Autodesk Fusion 360 part; units mm, degrees
(part 6 of 18)
  spline S29 degree 5 poles (33.0522, -6.0428) (33.0487, -6.0404) (33.0419, -6.0356) (33.0316, -6.0284) (33.018, -6.0188) (33.0009, -6.0069) (32.9839, -5.995) (32.9669, -5.9831) (32.9499, -5.9714) (32.9329, -5.9596) (32.9159, -5.948) (32.899, -5.9363) (32.8821, -5.9248) (32.8652, -5.9132) (32.8483, -5.9018) (32.8314, -5.8903) (32.8145, -5.879) (32.7977, -5.8676) (32.7809, -5.8563) (32.7641, -5.8451) (32.7473, -5.8339) (32.7306, -5.8228) (32.7138, -5.8117) (32.6971, -5.8007) (32.6804, -5.7897) (32.6637, -5.7788) (32.6471, -5.7679) (32.6305, -5.7571) (32.6139, -5.7463) (32.5973, -5.7356) (32.5807, -5.7249) (32.5642, -5.7143) (32.5476, -5.7037) (32.5311, -5.6932) (32.5147, -5.6827) (32.4982, -5.6723) (32.4818, -5.6619) (32.4654, -5.6516) (32.449, -5.6413) (32.4326, -5.6311) (32.4163, -5.6209) (32.4, -5.6108) (32.3837, -5.6007) (32.3675, -5.5907) (32.3512, -5.5807) (32.335, -5.5708) (32.3188, -5.5609) (32.3027, -5.5511) (32.2865, -5.5414) (32.2704, -5.5316) (32.2544, -5.522) (32.2383, -5.5123) (32.2223, -5.5028) (32.2063, -5.4933) (32.1903, -5.4838) (32.1744, -5.4744) (32.1585, -5.465) (32.1426, -5.4557) (32.1267, -5.4464) (32.1109, -5.4372) (32.0951, -5.4281) (32.0793, -5.419) (32.0636, -5.4099) (32.0479, -5.4009) (32.0322, -5.3919) (32.0166, -5.383) (32.0009, -5.3742) (31.9854, -5.3654) (31.9698, -5.3566) (31.9543, -5.3479) (31.9388, -5.3393) (31.9233, -5.3307) (31.9079, -5.3221) (31.8925, -5.3136) (31.8771, -5.3052) (31.8618, -5.2968) (31.8465, -5.2884) (31.8313, -5.2801) (31.816, -5.2719) (31.8008, -5.2637) (31.7857, -5.2555) (31.7706, -5.2474) (31.7555, -5.2394) (31.7404, -5.2314) (31.7254, -5.2235) (31.7104, -5.2156) (31.6955, -5.2077) (31.6806, -5.2) (31.6657, -5.1922) (31.6509, -5.1845) (31.6361, -5.1769) (31.6213, -5.1693) (31.6066, -5.1618) (31.5919, -5.1543) (31.5773, -5.1469) (31.5627, -5.1395) (31.5481, -5.1322) (31.5336, -5.1249) (31.5191, -5.1177) (31.5047, -5.1105) (31.4903, -5.1034) (31.4759, -5.0963) (31.4616, -5.0893) (31.4474, -5.0823) (31.4331, -5.0754) (31.419, -5.0686) (31.4048, -5.0617) (31.3907, -5.055) (31.3767, -5.0483) (31.3627, -5.0416) (31.3487, -5.035) (31.3348, -5.0284) (31.3209, -5.0219) (31.3071, -5.0155) (31.2933, -5.0091) (31.2796, -5.0027) (31.2659, -4.9964) (31.2522, -4.9902) (31.2387, -4.984) (31.2251, -4.9778) (31.2116, -4.9717) (31.1982, -4.9657) (31.1848, -4.9597) (31.1714, -4.9537) (31.1582, -4.9478) (31.1449, -4.942) (31.1317, -4.9362) (31.1186, -4.9305) (31.1055, -4.9248) (31.0925, -4.9191) (31.0795, -4.9136) (31.0666, -4.908) (31.0537, -4.9025) (31.0409, -4.8971) (31.0281, -4.8917) (31.0154, -4.8864) (31.0028, -4.8811) (30.9902, -4.8759) (30.9777, -4.8707) (30.9652, -4.8656) (30.9528, -4.8605) (30.9405, -4.8555) (30.9282, -4.8505) (30.9159, -4.8456) (30.9038, -4.8407) (30.8916, -4.8359) (30.8796, -4.8311) (30.8676, -4.8264) (30.8557, -4.8217) (30.8438, -4.8171) (30.832, -4.8126) (30.8203, -4.808) (30.8086, -4.8036) (30.797, -4.7992) (30.7855, -4.7948) (30.774, -4.7905) (30.7626, -4.7862) (30.7513, -4.782) (30.7401, -4.7779) (30.7289, -4.7738) (30.7178, -4.7697) (30.7067, -4.7657) (30.6957, -4.7617) (30.6848, -4.7578) (30.674, -4.754) (30.6633, -4.7502) (30.6526, -4.7464) (30.642, -4.7427) (30.6315, -4.7391) (30.621, -4.7354) (30.6106, -4.7319) (30.6004, -4.7284) (30.5901, -4.7249) (30.58, -4.7215) (30.57, -4.7182) (30.56, -4.7149) (30.5501, -4.7116) (30.5403, -4.7084) (30.5306, -4.7053) (30.521, -4.7022) (30.5115, -4.6991) (30.502, -4.6961) (30.4926, -4.6932) (30.4834, -4.6903) (30.4742, -4.6874) (30.4651, -4.6846) (30.4561, -4.6818) (30.4472, -4.6791) (30.4384, -4.6765) (30.4297, -4.6739) (30.4211, -4.6713) (30.4126, -4.6688) (30.4042, -4.6663) (30.3958, -4.6639) (30.3876, -4.6616) (30.3795, -4.6593) (30.3715, -4.657) (30.3636, -4.6548) (30.3559, -4.6526) (30.3482, -4.6505) (30.3406, -4.6484) (30.3332, -4.6464) (30.3258, -4.6444) (30.3186, -4.6425) (30.3115, -4.6407) (30.3045, -4.6388) (30.2976, -4.637) (30.2909, -4.6353) (30.2842, -4.6336) (30.2777, -4.632) (30.2713, -4.6304) (30.2651, -4.6289) (30.259, -4.6274) (30.253, -4.6259) (30.2471, -4.6245) (30.2414, -4.6232) (30.2358, -4.6219) (30.2304, -4.6206) (30.2251, -4.6194) (30.22, -4.6182) (30.215, -4.6171) (30.2101, -4.6161) (30.2054, -4.615) (30.2009, -4.614) (30.1965, -4.6131) (30.1923, -4.6122) (30.1882, -4.6114) (30.1843, -4.6106) (30.1806, -4.6098) (30.1771, -4.6091) (30.1737, -4.6084) (30.1705, -4.6078) (30.1675, -4.6072) (30.1647, -4.6067) (30.162, -4.6062) (30.1596, -4.6058) (30.1574, -4.6054) (30.1553, -4.605) (30.1535, -4.6047) (30.1519, -4.6044) (30.1505, -4.6042) (30.1496, -4.604) (30.149, -4.6039) (30.1487, -4.6039) (30.1485, -4.6039) knots -1 -1 -1 -1 -1 -1 -0.99583333 -0.99166667 -0.9875 -0.98333333 -0.97916667 -0.975 -0.97083333 -0.96666667 -0.9625 -0.95833333 -0.95416667 -0.95 -0.94583333 -0.94166667 -0.9375 -0.93333333 -0.92916667 -0.925 -0.92083333 -0.91666667 -0.9125 -0.90833333 -0.90416667 -0.9 -0.89583333 -0.89166667 -0.8875 -0.88333333 -0.87916667 -0.875 -0.87083333 -0.86666667 -0.8625 -0.85833333 -0.85416667 -0.85 -0.84583333 -0.84166667 -0.8375 -0.83333333 -0.82916667 -0.825 -0.82083333 -0.81666667 -0.8125 -0.80833333 -0.80416667 -0.8 -0.79583333 -0.79166667 -0.7875 -0.78333333 -0.77916667 -0.775 -0.77083333 -0.76666667 -0.7625 -0.75833333 -0.75416667 -0.75 -0.74583333 -0.74166667 -0.7375 -0.73333333 -0.72916667 -0.725 -0.72083333 -0.71666667 -0.7125 -0.70833333 -0.70416667 -0.7 -0.69583333 -0.69166667 -0.6875 -0.68333333 -0.67916667 -0.675 -0.67083333 -0.66666667 -0.6625 -0.65833333 -0.65416667 -0.65 -0.64583333 -0.64166667 -0.6375 -0.63333333 -0.62916667 -0.625 -0.62083333 -0.61666667 -0.6125 -0.60833333 -0.60416667 -0.6 -0.59583333 -0.59166667 -0.5875 -0.58333333 -0.57916667 -0.575 -0.57083333 -0.56666667 -0.5625 -0.55833333 -0.55416667 -0.55 -0.54583333 -0.54166667 -0.5375 -0.53333333 -0.52916667 -0.525 -0.52083333 -0.51666667 -0.5125 -0.50833333 -0.50416667 -0.5 -0.49583333 -0.49166667 -0.4875 -0.48333333 -0.47916667 -0.475 -0.47083333 -0.46666667 -0.4625 -0.45833333 -0.45416667 -0.45 -0.44583333 -0.44166667 -0.4375 -0.43333333 -0.42916667 -0.425 -0.42083333 -0.41666667 -0.4125 -0.40833333 -0.40416667 -0.4 -0.39583333 -0.39166667 -0.3875 -0.38333333 -0.37916667 -0.375 -0.37083333 -0.36666667 -0.3625 -0.35833333 -0.35416667 -0.35 -0.34583333 -0.34166667 -0.3375 -0.33333333 -0.32916667 -0.325 -0.32083333 -0.31666667 -0.3125 -0.30833333 -0.30416667 -0.3 -0.29583333 -0.29166667 -0.2875 -0.28333333 -0.27916667 -0.275 -0.27083333 -0.26666667 -0.2625 -0.25833333 -0.25416667 -0.25 -0.24583333 -0.24166667 -0.2375 -0.23333333 -0.22916667 -0.225 -0.22083333 -0.21666667 -0.2125 -0.20833333 -0.20416667 -0.2 -0.19583333 -0.19166667 -0.1875 -0.18333333 -0.17916667 -0.175 -0.17083333 -0.16666667 -0.1625 -0.15833333 -0.15416667 -0.15 -0.14583333 -0.14166667 -0.1375 -0.13333333 -0.12916667 -0.125 -0.12083333 -0.11666667 -0.1125 -0.10833333 -0.10416667 -0.1 -0.09583333 -0.09166667 -0.0875 -0.08333333 -0.07916667 -0.075 -0.07083333 -0.06666667 -0.0625 -0.05833333 -0.05416667 -0.05 -0.04583333 -0.04166667 -0.0375 -0.03333333 -0.02916667 -0.025 -0.02083333 -0.01666667 -0.0125 -0.00833333 -0.00416667 0 0 0 0 0 0
  line L58 (30.1485, -4.6039) -> (30.1472, -4.6036)
  line L59 (30.1472, -4.6036) -> (28.5441, -4.3588)
  arc A30 (28.5441, -4.3588) -> (28.8266, -1.6711) centre (0, 0) ccw
  line L60 (28.8266, -1.6711) -> (30.4455, -1.7649)
  line L61 (30.4455, -1.7649) -> (30.4469, -1.765)
  spline S30 degree 5 poles (30.4469, -1.765) (30.4471, -1.765) (30.4474, -1.765) (30.448, -1.765) (30.449, -1.7651) (30.4503, -1.7651) (30.452, -1.7652) (30.4538, -1.7653) (30.4559, -1.7653) (30.4581, -1.7654) (30.4606, -1.7655) (30.4633, -1.7655) (30.4662, -1.7656) (30.4692, -1.7657) (30.4725, -1.7657) (30.4759, -1.7658) (30.4795, -1.7658) (30.4833, -1.7658) (30.4873, -1.7659) (30.4914, -1.7659) (30.4958, -1.7659) (30.5002, -1.7659) (30.5049, -1.7659) (30.5097, -1.7659) (30.5147, -1.7658) (30.5198, -1.7658) (30.5251, -1.7657) (30.5305, -1.7656) (30.5361, -1.7655) (30.5418, -1.7654) (30.5477, -1.7653) (30.5537, -1.7651) (30.5598, -1.7649) (30.5661, -1.7647) (30.5726, -1.7645) (30.5791, -1.7643) (30.5858, -1.7641) (30.5927, -1.7638) (30.5996, -1.7635) (30.6067, -1.7632) (30.6139, -1.7629) (30.6213, -1.7625) (30.6288, -1.7621) (30.6363, -1.7617) (30.6441, -1.7613) (30.6519, -1.7609) (30.6598, -1.7604) (30.6679, -1.7599) (30.6761, -1.7594) (30.6844, -1.7588) (30.6928, -1.7582) (30.7013, -1.7576) (30.7099, -1.757) (30.7187, -1.7563) (30.7275, -1.7557) (30.7365, -1.755) (30.7455, -1.7542) (30.7547, -1.7534) (30.764, -1.7527) (30.7734, -1.7518) (30.7828, -1.751) (30.7924, -1.7501) (30.8021, -1.7492) (30.8118, -1.7482) (30.8217, -1.7473) (30.8317, -1.7463) (30.8417, -1.7452) (30.8519, -1.7442) (30.8621, -1.7431) (30.8725, -1.7419) (30.8829, -1.7408) (30.8934, -1.7396) (30.904, -1.7384) (30.9148, -1.7371) (30.9255, -1.7358) (30.9364, -1.7345) (30.9474, -1.7331) (30.9584, -1.7318) (30.9696, -1.7303) (30.9808, -1.7289) (30.9921, -1.7274) (31.0035, -1.7259) (31.015, -1.7243) (31.0265, -1.7227) (31.0382, -1.7211) (31.0499, -1.7195) (31.0617, -1.7178) (31.0736, -1.716) (31.0855, -1.7143) (31.0976, -1.7125) (31.1097, -1.7106) (31.1219, -1.7088) (31.1341, -1.7069) (31.1465, -1.7049) (31.1589, -1.7029) (31.1714, -1.7009) (31.1839, -1.6989) (31.1965, -1.6968) (31.2092, -1.6947) (31.222, -1.6925) (31.2349, -1.6903) (31.2478, -1.6881) (31.2608, -1.6858) (31.2738, -1.6835) (31.287, -1.6812) (31.3002, -1.6788) (31.3134, -1.6763) (31.3268, -1.6739) (31.3402, -1.6714) (31.3536, -1.6689) (31.3672, -1.6663) (31.3808, -1.6637) (31.3944, -1.661) (31.4081, -1.6583) (31.4219, -1.6556) (31.4358, -1.6528) (31.4497, -1.65) (31.4637, -1.6472) (31.4777, -1.6443) (31.4918, -1.6414) (31.506, -1.6384) (31.5202, -1.6354) (31.5345, -1.6324) (31.5488, -1.6293) (31.5632, -1.6262) (31.5777, -1.623) (31.5922, -1.6198) (31.6068, -1.6166) (31.6215, -1.6133) (31.6362, -1.61) (31.6509, -1.6066) (31.6657, -1.6032) (31.6806, -1.5998) (31.6955, -1.5963) (31.7105, -1.5928) (31.7255, -1.5892) (31.7406, -1.5856) (31.7557, -1.582) (31.7709, -1.5783) (31.7862, -1.5746) (31.8015, -1.5708) (31.8168, -1.567) (31.8322, -1.5632) (31.8477, -1.5593) (31.8632, -1.5553) (31.8788, -1.5514) (31.8944, -1.5473) (31.9101, -1.5433) (31.9258, -1.5392) (31.9415, -1.5351) (31.9573, -1.5309) (31.9732, -1.5267) (31.9891, -1.5224) (32.0051, -1.5181) (32.0211, -1.5137) (32.0372, -1.5093) (32.0533, -1.5049) (32.0694, -1.5004) (32.0856, -1.4959) (32.1019, -1.4914) (32.1181, -1.4868) (32.1345, -1.4821) (32.1509, -1.4774) (32.1673, -1.4727) (32.1838, -1.4679) (32.2003, -1.4631) (32.2169, -1.4583) (32.2335, -1.4534) (32.2501, -1.4484) (32.2668, -1.4434) (32.2836, -1.4384) (32.3003, -1.4333) (32.3172, -1.4282) (32.334, -1.4231) (32.3509, -1.4179) (32.3679, -1.4126) (32.3849, -1.4073) (32.4019, -1.402) (32.419, -1.3966) (32.4361, -1.3912) (32.4533, -1.3858) (32.4705, -1.3803) (32.4877, -1.3747) (32.505, -1.3691) (32.5223, -1.3635) (32.5397, -1.3578) (32.5571, -1.3521) (32.5745, -1.3463) (32.592, -1.3405) (32.6095, -1.3347) (32.627, -1.3288) (32.6446, -1.3228) (32.6622, -1.3169) (32.6799, -1.3108) (32.6976, -1.3048) (32.7153, -1.2986) (32.7331, -1.2925) (32.7509, -1.2863) (32.7688, -1.28) (32.7867, -1.2738) (32.8046, -1.2674) (32.8225, -1.261) (32.8405, -1.2546) (32.8585, -1.2482) (32.8766, -1.2416) (32.8947, -1.2351) (32.9128, -1.2285) (32.931, -1.2218) (32.9492, -1.2152) (32.9674, -1.2084) (32.9856, -1.2016) (33.0039, -1.1948) (33.0223, -1.188) (33.0406, -1.181) (33.059, -1.1741) (33.0774, -1.1671) (33.0959, -1.16) (33.1144, -1.153) (33.1329, -1.1458) (33.1514, -1.1387) (33.17, -1.1314) (33.1886, -1.1242) (33.2073, -1.1168) (33.2259, -1.1095) (33.2447, -1.1021) (33.2634, -1.0946) (33.2821, -1.0872) (33.3009, -1.0796) (33.3198, -1.072) (33.3386, -1.0644) (33.3575, -1.0567) (33.3764, -1.049) (33.3953, -1.0413) (33.4143, -1.0335) (33.4333, -1.0256) (33.4523, -1.0177) (33.4714, -1.0098) (33.4904, -1.0018) (33.5096, -0.9938) (33.5287, -0.9857) (33.5478, -0.9776) (33.5632, -0.971) (33.5747, -0.9661) (33.5824, -0.9628) (33.5862, -0.9612) knots 0 0 0 0 0 0 0.00416667 0.00833333 0.0125 0.01666667 0.02083333 0.025 0.02916667 0.03333333 0.0375 0.04166667 0.04583333 0.05 0.05416667 0.05833333 0.0625 0.06666667 0.07083333 0.075 0.07916667 0.08333333 0.0875 0.09166667 0.09583333 0.1 0.10416667 0.10833333 0.1125 0.11666667 0.12083333 0.125 0.12916667 0.13333333 0.1375 0.14166667 0.14583333 0.15 0.15416667 0.15833333 0.1625 0.16666667 0.17083333 0.175 0.17916667 0.18333333 0.1875 0.19166667 0.19583333 0.2 0.20416667 0.20833333 0.2125 0.21666667 0.22083333 0.225 0.22916667 0.23333333 0.2375 0.24166667 0.24583333 0.25 0.25416667 0.25833333 0.2625 0.26666667 0.27083333 0.275 0.27916667 0.28333333 0.2875 0.29166667 0.29583333 0.3 0.30416667 0.30833333 0.3125 0.31666667 0.32083333 0.325 0.32916667 0.33333333 0.3375 0.34166667 0.34583333 0.35 0.35416667 0.35833333 0.3625 0.36666667 0.37083333 0.375 0.37916667 0.38333333 0.3875 0.39166667 0.39583333 0.4 0.40416667 0.40833333 0.4125 0.41666667 0.42083333 0.425 0.42916667 0.43333333 0.4375 0.44166667 0.44583333 0.45 0.45416667 0.45833333 0.4625 0.46666667 0.47083333 0.475 0.47916667 0.48333333 0.4875 0.49166667 0.49583333 0.5 0.50416667 0.50833333 0.5125 0.51666667 0.52083333 0.525 0.52916667 0.53333333 0.5375 0.54166667 0.54583333 0.55 0.55416667 0.55833333 0.5625 0.56666667 0.57083333 0.575 0.57916667 0.58333333 0.5875 0.59166667 0.59583333 0.6 0.60416667 0.60833333 0.6125 0.61666667 0.62083333 0.625 0.62916667 0.63333333 0.6375 0.64166667 0.64583333 0.65 0.65416667 0.65833333 0.6625 0.66666667 0.67083333 0.675 0.67916667 0.68333333 0.6875 0.69166667 0.69583333 0.7 0.70416667 0.70833333 0.7125 0.71666667 0.72083333 0.725 0.72916667 0.73333333 0.7375 0.74166667 0.74583333 0.75 0.75416667 0.75833333 0.7625 0.76666667 0.77083333 0.775 0.77916667 0.78333333 0.7875 0.79166667 0.79583333 0.8 0.80416667 0.80833333 0.8125 0.81666667 0.82083333 0.825 0.82916667 0.83333333 0.8375 0.84166667 0.84583333 0.85 0.85416667 0.85833333 0.8625 0.86666667 0.87083333 0.875 0.87916667 0.88333333 0.8875 0.89166667 0.89583333 0.9 0.90416667 0.90833333 0.9125 0.91666667 0.92083333 0.925 0.92916667 0.93333333 0.9375 0.94166667 0.94583333 0.95 0.95416667 0.95833333 0.9625 0.96666667 0.97083333 0.975 0.97916667 0.98333333 0.9875 0.99166667 0.99583333 1 1 1 1 1 1
  arc A31 (33.5862, -0.9612) -> (33.5862, 0.9612) centre (0, 0) ccw
  spline S31 degree 5 poles (33.5862, 0.9612) (33.5824, 0.9628) (33.5747, 0.9661) (33.5632, 0.971) (33.5478, 0.9776) (33.5287, 0.9857) (33.5096, 0.9938) (33.4904, 1.0018) (33.4714, 1.0098) (33.4523, 1.0177) (33.4333, 1.0256) (33.4143, 1.0335) (33.3953, 1.0413) (33.3764, 1.049) (33.3575, 1.0567) (33.3386, 1.0644) (33.3198, 1.072) (33.3009, 1.0796) (33.2821, 1.0872) (33.2634, 1.0946) (33.2447, 1.1021) (33.2259, 1.1095) (33.2073, 1.1168) (33.1886, 1.1242) (33.17, 1.1314) (33.1514, 1.1387) (33.1329, 1.1458) (33.1144, 1.153) (33.0959, 1.16) (33.0774, 1.1671) (33.059, 1.1741) (33.0406, 1.181) (33.0223, 1.188) (33.0039, 1.1948) (32.9856, 1.2016) (32.9674, 1.2084) (32.9492, 1.2152) (32.931, 1.2218) (32.9128, 1.2285) (32.8947, 1.2351) (32.8766, 1.2416) (32.8585, 1.2482) (32.8405, 1.2546) (32.8225, 1.261) (32.8046, 1.2674) (32.7867, 1.2738) (32.7688, 1.28) (32.7509, 1.2863) (32.7331, 1.2925) (32.7153, 1.2986) (32.6976, 1.3048) (32.6799, 1.3108) (32.6622, 1.3169) (32.6446, 1.3228) (32.627, 1.3288) (32.6095, 1.3347) (32.592, 1.3405) (32.5745, 1.3463) (32.5571, 1.3521) (32.5397, 1.3578) (32.5223, 1.3635) (32.505, 1.3691) (32.4877, 1.3747) (32.4705, 1.3803) (32.4533, 1.3858) (32.4361, 1.3912) (32.419, 1.3966) (32.4019, 1.402) (32.3849, 1.4073) (32.3679, 1.4126) (32.3509, 1.4179) (32.334, 1.4231) (32.3172, 1.4282) (32.3003, 1.4333) (32.2836, 1.4384) (32.2668, 1.4434) (32.2501, 1.4484) (32.2335, 1.4534) (32.2169, 1.4583) (32.2003, 1.4631) (32.1838, 1.4679) (32.1673, 1.4727) (32.1509, 1.4774) (32.1345, 1.4821) (32.1181, 1.4868) (32.1019, 1.4914) (32.0856, 1.4959) (32.0694, 1.5004) (32.0533, 1.5049) (32.0372, 1.5093) (32.0211, 1.5137) (32.0051, 1.5181) (31.9891, 1.5224) (31.9732, 1.5267) (31.9573, 1.5309) (31.9415, 1.5351) (31.9258, 1.5392) (31.9101, 1.5433) (31.8944, 1.5473) (31.8788, 1.5514) (31.8632, 1.5553) (31.8477, 1.5593) (31.8322, 1.5632) (31.8168, 1.567) (31.8015, 1.5708) (31.7862, 1.5746) (31.7709, 1.5783) (31.7557, 1.582) (31.7406, 1.5856) (31.7255, 1.5892) (31.7105, 1.5928) (31.6955, 1.5963) (31.6806, 1.5998) (31.6657, 1.6032) (31.6509, 1.6066) (31.6362, 1.61) (31.6215, 1.6133) (31.6068, 1.6166) (31.5922, 1.6198) (31.5777, 1.623) (31.5632, 1.6262) (31.5488, 1.6293) (31.5345, 1.6324) (31.5202, 1.6354) (31.506, 1.6384) (31.4918, 1.6414) (31.4777, 1.6443) (31.4637, 1.6472) (31.4497, 1.65) (31.4358, 1.6528) (31.4219, 1.6556) (31.4081, 1.6583) (31.3944, 1.661) (31.3808, 1.6637) (31.3672, 1.6663) (31.3536, 1.6689) (31.3402, 1.6714) (31.3268, 1.6739) (31.3134, 1.6763) (31.3002, 1.6788) (31.287, 1.6812) (31.2738, 1.6835) (31.2608, 1.6858) (31.2478, 1.6881) (31.2349, 1.6903) (31.222, 1.6925) (31.2092, 1.6947) (31.1965, 1.6968) (31.1839, 1.6989) (31.1714, 1.7009) (31.1589, 1.7029) (31.1465, 1.7049) (31.1341, 1.7069) (31.1219, 1.7088) (31.1097, 1.7106) (31.0976, 1.7125) (31.0855, 1.7143) (31.0736, 1.716) (31.0617, 1.7178) (31.0499, 1.7195) (31.0382, 1.7211) (31.0265, 1.7227) (31.015, 1.7243) (31.0035, 1.7259) (30.9921, 1.7274) (30.9808, 1.7289) (30.9696, 1.7303) (30.9584, 1.7318) (30.9474, 1.7331) (30.9364, 1.7345) (30.9255, 1.7358) (30.9148, 1.7371) (30.904, 1.7384) (30.8934, 1.7396) (30.8829, 1.7408) (30.8725, 1.7419) (30.8621, 1.7431) (30.8519, 1.7442) (30.8417, 1.7452) (30.8317, 1.7463) (30.8217, 1.7473) (30.8118, 1.7482) (30.8021, 1.7492) (30.7924, 1.7501) (30.7828, 1.751) (30.7734, 1.7518) (30.764, 1.7527) (30.7547, 1.7534) (30.7455, 1.7542) (30.7365, 1.755) (30.7275, 1.7557) (30.7187, 1.7563) (30.7099, 1.757) (30.7013, 1.7576) (30.6928, 1.7582) (30.6844, 1.7588) (30.6761, 1.7594) (30.6679, 1.7599) (30.6598, 1.7604) (30.6519, 1.7609) (30.6441, 1.7613) (30.6363, 1.7617) (30.6288, 1.7621) (30.6213, 1.7625) (30.6139, 1.7629) (30.6067, 1.7632) (30.5996, 1.7635) (30.5927, 1.7638) (30.5858, 1.7641) (30.5791, 1.7643) (30.5726, 1.7645) (30.5661, 1.7647) (30.5598, 1.7649) (30.5537, 1.7651) (30.5477, 1.7653) (30.5418, 1.7654) (30.5361, 1.7655) (30.5305, 1.7656) (30.5251, 1.7657) (30.5198, 1.7658) (30.5147, 1.7658) (30.5097, 1.7659) (30.5049, 1.7659) (30.5002, 1.7659) (30.4958, 1.7659) (30.4914, 1.7659) (30.4873, 1.7659) (30.4833, 1.7658) (30.4795, 1.7658) (30.4759, 1.7658) (30.4725, 1.7657) (30.4692, 1.7657) (30.4662, 1.7656) (30.4633, 1.7655) (30.4606, 1.7655) (30.4581, 1.7654) (30.4559, 1.7653) (30.4538, 1.7653) (30.452, 1.7652) (30.4503, 1.7651) (30.449, 1.7651) (30.448, 1.765) (30.4474, 1.765) (30.4471, 1.765) (30.4469, 1.765) knots -1 -1 -1 -1 -1 -1 -0.99583333 -0.99166667 -0.9875 -0.98333333 -0.97916667 -0.975 -0.97083333 -0.96666667 -0.9625 -0.95833333 -0.95416667 -0.95 -0.94583333 -0.94166667 -0.9375 -0.93333333 -0.92916667 -0.925 -0.92083333 -0.91666667 -0.9125 -0.90833333 -0.90416667 -0.9 -0.89583333 -0.89166667 -0.8875 -0.88333333 -0.87916667 -0.875 -0.87083333 -0.86666667 -0.8625 -0.85833333 -0.85416667 -0.85 -0.84583333 -0.84166667 -0.8375 -0.83333333 -0.82916667 -0.825 -0.82083333 -0.81666667 -0.8125 -0.80833333 -0.80416667 -0.8 -0.79583333 -0.79166667 -0.7875 -0.78333333 -0.77916667 -0.775 -0.77083333 -0.76666667 -0.7625 -0.75833333 -0.75416667 -0.75 -0.74583333 -0.74166667 -0.7375 -0.73333333 -0.72916667 -0.725 -0.72083333 -0.71666667 -0.7125 -0.70833333 -0.70416667 -0.7 -0.69583333 -0.69166667 -0.6875 -0.68333333 -0.67916667 -0.675 -0.67083333 -0.66666667 -0.6625 -0.65833333 -0.65416667 -0.65 -0.64583333 -0.64166667 -0.6375 -0.63333333 -0.62916667 -0.625 -0.62083333 -0.61666667 -0.6125 -0.60833333 -0.60416667 -0.6 -0.59583333 -0.59166667 -0.5875 -0.58333333 -0.57916667 -0.575 -0.57083333 -0.56666667 -0.5625 -0.55833333 -0.55416667 -0.55 -0.54583333 -0.54166667 -0.5375 -0.53333333 -0.52916667 -0.525 -0.52083333 -0.51666667 -0.5125 -0.50833333 -0.50416667 -0.5 -0.49583333 -0.49166667 -0.4875 -0.48333333 -0.47916667 -0.475 -0.47083333 -0.46666667 -0.4625 -0.45833333 -0.45416667 -0.45 -0.44583333 -0.44166667 -0.4375 -0.43333333 -0.42916667 -0.425 -0.42083333 -0.41666667 -0.4125 -0.40833333 -0.40416667 -0.4 -0.39583333 -0.39166667 -0.3875 -0.38333333 -0.37916667 -0.375 -0.37083333 -0.36666667 -0.3625 -0.35833333 -0.35416667 -0.35 -0.34583333 -0.34166667 -0.3375 -0.33333333 -0.32916667 -0.325 -0.32083333 -0.31666667 -0.3125 -0.30833333 -0.30416667 -0.3 -0.29583333 -0.29166667 -0.2875 -0.28333333 -0.27916667 -0.275 -0.27083333 -0.26666667 -0.2625 -0.25833333 -0.25416667 -0.25 -0.24583333 -0.24166667 -0.2375 -0.23333333 -0.22916667 -0.225 -0.22083333 -0.21666667 -0.2125 -0.20833333 -0.20416667 -0.2 -0.19583333 -0.19166667 -0.1875 -0.18333333 -0.17916667 -0.175 -0.17083333 -0.16666667 -0.1625 -0.15833333 -0.15416667 -0.15 -0.14583333 -0.14166667 -0.1375 -0.13333333 -0.12916667 -0.125 -0.12083333 -0.11666667 -0.1125 -0.10833333 -0.10416667 -0.1 -0.09583333 -0.09166667 -0.0875 -0.08333333 -0.07916667 -0.075 -0.07083333 -0.06666667 -0.0625 -0.05833333 -0.05416667 -0.05 -0.04583333 -0.04166667 -0.0375 -0.03333333 -0.02916667 -0.025 -0.02083333 -0.01666667 -0.0125 -0.00833333 -0.00416667 0 0 0 0 0 0
  line L62 (30.4469, 1.765) -> (30.4455, 1.7649)
  line L63 (30.4455, 1.7649) -> (28.8266, 1.6711)
  arc A32 (28.8266, 1.6711) -> (28.5441, 4.3588) centre (0, 0) ccw
  line L64 (28.5441, 4.3588) -> (30.1472, 4.6036)
  line L65 (30.1472, 4.6036) -> (30.1485, 4.6039)
  spline S32 degree 5 poles (30.1485, 4.6039) (30.1487, 4.6039) (30.149, 4.6039) (30.1496, 4.604) (30.1505, 4.6042) (30.1519, 4.6044) (30.1535, 4.6047) (30.1553, 4.605) (30.1574, 4.6054) (30.1596, 4.6058) (30.162, 4.6062) (30.1647, 4.6067) (30.1675, 4.6072) (30.1705, 4.6078) (30.1737, 4.6084) (30.1771, 4.6091) (30.1806, 4.6098) (30.1843, 4.6106) (30.1882, 4.6114) (30.1923, 4.6122) (30.1965, 4.6131) (30.2009, 4.614) (30.2054, 4.615) (30.2101, 4.6161) (30.215, 4.6171) (30.22, 4.6182) (30.2251, 4.6194) (30.2304, 4.6206) (30.2358, 4.6219) (30.2414, 4.6232) (30.2471, 4.6245) (30.253, 4.6259) (30.259, 4.6274) (30.2651, 4.6289) (30.2713, 4.6304) (30.2777, 4.632) (30.2842, 4.6336) (30.2909, 4.6353) (30.2976, 4.637) (30.3045, 4.6388) (30.3115, 4.6407) (30.3186, 4.6425) (30.3258, 4.6444) (30.3332, 4.6464) (30.3406, 4.6484) (30.3482, 4.6505) (30.3559, 4.6526) (30.3636, 4.6548) (30.3715, 4.657) (30.3795, 4.6593) (30.3876, 4.6616) (30.3958, 4.6639) (30.4042, 4.6663) (30.4126, 4.6688) (30.4211, 4.6713) (30.4297, 4.6739) (30.4384, 4.6765) (30.4472, 4.6791) (30.4561, 4.6818) (30.4651, 4.6846) (30.4742, 4.6874) (30.4834, 4.6903) (30.4926, 4.6932) (30.502, 4.6961) (30.5115, 4.6991) (30.521, 4.7022) (30.5306, 4.7053) (30.5403, 4.7084) (30.5501, 4.7116) (30.56, 4.7149) (30.57, 4.7182) (30.58, 4.7215) (30.5901, 4.7249) (30.6004, 4.7284) (30.6106, 4.7319) (30.621, 4.7354) (30.6315, 4.7391) (30.642, 4.7427) (30.6526, 4.7464) (30.6633, 4.7502) (30.674, 4.754) (30.6848, 4.7578) (30.6957, 4.7617) (30.7067, 4.7657) (30.7178, 4.7697) (30.7289, 4.7738) (30.7401, 4.7779) (30.7513, 4.782) (30.7626, 4.7862) (30.774, 4.7905) (30.7855, 4.7948) (30.797, 4.7992) (30.8086, 4.8036) (30.8203, 4.808) (30.832, 4.8126) (30.8438, 4.8171) (30.8557, 4.8217) (30.8676, 4.8264) (30.8796, 4.8311) (30.8916, 4.8359) (30.9038, 4.8407) (30.9159, 4.8456) (30.9282, 4.8505) (30.9405, 4.8555) (30.9528, 4.8605) (30.9652, 4.8656) (30.9777, 4.8707) (30.9902, 4.8759) (31.0028, 4.8811) (31.0154, 4.8864) (31.0281, 4.8917) (31.0409, 4.8971) (31.0537, 4.9025) (31.0666, 4.908) (31.0795, 4.9136) (31.0925, 4.9191) (31.1055, 4.9248) (31.1186, 4.9305) (31.1317, 4.9362) (31.1449, 4.942) (31.1582, 4.9478) (31.1714, 4.9537) (31.1848, 4.9597) (31.1982, 4.9657) (31.2116, 4.9717) (31.2251, 4.9778) (31.2387, 4.984) (31.2522, 4.9902) (31.2659, 4.9964) (31.2796, 5.0027) (31.2933, 5.0091) (31.3071, 5.0155) (31.3209, 5.0219) (31.3348, 5.0284) (31.3487, 5.035) (31.3627, 5.0416) (31.3767, 5.0483) (31.3907, 5.055) (31.4048, 5.0617) (31.419, 5.0686) (31.4331, 5.0754) (31.4474, 5.0823) (31.4616, 5.0893) (31.4759, 5.0963) (31.4903, 5.1034) (31.5047, 5.1105) (31.5191, 5.1177) (31.5336, 5.1249) (31.5481, 5.1322) (31.5627, 5.1395) (31.5773, 5.1469) (31.5919, 5.1543) (31.6066, 5.1618) (31.6213, 5.1693) (31.6361, 5.1769) (31.6509, 5.1845) (31.6657, 5.1922) (31.6806, 5.2) (31.6955, 5.2077) (31.7104, 5.2156) (31.7254, 5.2235) (31.7404, 5.2314) (31.7555, 5.2394) (31.7706, 5.2474) (31.7857, 5.2555) (31.8008, 5.2637) (31.816, 5.2719) (31.8313, 5.2801) (31.8465, 5.2884) (31.8618, 5.2968) (31.8771, 5.3052) (31.8925, 5.3136) (31.9079, 5.3221) (31.9233, 5.3307) (31.9388, 5.3393) (31.9543, 5.3479) (31.9698, 5.3566) (31.9854, 5.3654) (32.0009, 5.3742) (32.0166, 5.383) (32.0322, 5.3919) (32.0479, 5.4009) (32.0636, 5.4099) (32.0793, 5.419) (32.0951, 5.4281) (32.1109, 5.4372) (32.1267, 5.4464) (32.1426, 5.4557) (32.1585, 5.465) (32.1744, 5.4744) (32.1903, 5.4838) (32.2063, 5.4933) (32.2223, 5.5028) (32.2383, 5.5123) (32.2544, 5.522) (32.2704, 5.5316) (32.2865, 5.5414) (32.3027, 5.5511) (32.3188, 5.5609) (32.335, 5.5708) (32.3512, 5.5807) (32.3675, 5.5907) (32.3837, 5.6007) (32.4, 5.6108) (32.4163, 5.6209) (32.4326, 5.6311) (32.449, 5.6413) (32.4654, 5.6516) (32.4818, 5.6619) (32.4982, 5.6723) (32.5147, 5.6827) (32.5311, 5.6932) (32.5476, 5.7037) (32.5642, 5.7143) (32.5807, 5.7249) (32.5973, 5.7356) (32.6139, 5.7463) (32.6305, 5.7571) (32.6471, 5.7679) (32.6637, 5.7788) (32.6804, 5.7897) (32.6971, 5.8007) (32.7138, 5.8117) (32.7306, 5.8228) (32.7473, 5.8339) (32.7641, 5.8451) (32.7809, 5.8563) (32.7977, 5.8676) (32.8145, 5.879) (32.8314, 5.8903) (32.8483, 5.9018) (32.8652, 5.9132) (32.8821, 5.9248) (32.899, 5.9363) (32.9159, 5.948) (32.9329, 5.9596) (32.9499, 5.9714) (32.9669, 5.9831) (32.9839, 5.995) (33.0009, 6.0069) (33.018, 6.0188) (33.0316, 6.0284) (33.0419, 6.0356) (33.0487, 6.0404) (33.0522, 6.0428) knots 0 0 0 0 0 0 0.00416667 0.00833333 0.0125 0.01666667 0.02083333 0.025 0.02916667 0.03333333 0.0375 0.04166667 0.04583333 0.05 0.05416667 0.05833333 0.0625 0.06666667 0.07083333 0.075 0.07916667 0.08333333 0.0875 0.09166667 0.09583333 0.1 0.10416667 0.10833333 0.1125 0.11666667 0.12083333 0.125 0.12916667 0.13333333 0.1375 0.14166667 0.14583333 0.15 0.15416667 0.15833333 0.1625 0.16666667 0.17083333 0.175 0.17916667 0.18333333 0.1875 0.19166667 0.19583333 0.2 0.20416667 0.20833333 0.2125 0.21666667 0.22083333 0.225 0.22916667 0.23333333 0.2375 0.24166667 0.24583333 0.25 0.25416667 0.25833333 0.2625 0.26666667 0.27083333 0.275 0.27916667 0.28333333 0.2875 0.29166667 0.29583333 0.3 0.30416667 0.30833333 0.3125 0.31666667 0.32083333 0.325 0.32916667 0.33333333 0.3375 0.34166667 0.34583333 0.35 0.35416667 0.35833333 0.3625 0.36666667 0.37083333 0.375 0.37916667 0.38333333 0.3875 0.39166667 0.39583333 0.4 0.40416667 0.40833333 0.4125 0.41666667 0.42083333 0.425 0.42916667 0.43333333 0.4375 0.44166667 0.44583333 0.45 0.45416667 0.45833333 0.4625 0.46666667 0.47083333 0.475 0.47916667 0.48333333 0.4875 0.49166667 0.49583333 0.5 0.50416667 0.50833333 0.5125 0.51666667 0.52083333 0.525 0.52916667 0.53333333 0.5375 0.54166667 0.54583333 0.55 0.55416667 0.55833333 0.5625 0.56666667 0.57083333 0.575 0.57916667 0.58333333 0.5875 0.59166667 0.59583333 0.6 0.60416667 0.60833333 0.6125 0.61666667 0.62083333 0.625 0.62916667 0.63333333 0.6375 0.64166667 0.64583333 0.65 0.65416667 0.65833333 0.6625 0.66666667 0.67083333 0.675 0.67916667 0.68333333 0.6875 0.69166667 0.69583333 0.7 0.70416667 0.70833333 0.7125 0.71666667 0.72083333 0.725 0.72916667 0.73333333 0.7375 0.74166667 0.74583333 0.75 0.75416667 0.75833333 0.7625 0.76666667 0.77083333 0.775 0.77916667 0.78333333 0.7875 0.79166667 0.79583333 0.8 0.80416667 0.80833333 0.8125 0.81666667 0.82083333 0.825 0.82916667 0.83333333 0.8375 0.84166667 0.84583333 0.85 0.85416667 0.85833333 0.8625 0.86666667 0.87083333 0.875 0.87916667 0.88333333 0.8875 0.89166667 0.89583333 0.9 0.90416667 0.90833333 0.9125 0.91666667 0.92083333 0.925 0.92916667 0.93333333 0.9375 0.94166667 0.94583333 0.95 0.95416667 0.95833333 0.9625 0.96666667 0.97083333 0.975 0.97916667 0.98333333 0.9875 0.99166667 0.99583333 1 1 1 1 1 1
  arc A33 (33.0522, 6.0428) -> (32.6525, 7.9232) centre (0, 0) ccw
  spline S33 degree 5 poles (32.6525, 7.9232) (32.6484, 7.924) (32.6402, 7.9256) (32.6279, 7.928) (32.6115, 7.9312) (32.5911, 7.9352) (32.5707, 7.9391) (32.5503, 7.943) (32.53, 7.9468) (32.5097, 7.9506) (32.4895, 7.9544) (32.4693, 7.9581) (32.4491, 7.9618) (32.4289, 7.9655) (32.4088, 7.9691) (32.3888, 7.9726) (32.3688, 7.9762) (32.3488, 7.9797) (32.3288, 7.9831) (32.3089, 7.9866) (32.289, 7.99) (32.2692, 7.9933) (32.2494, 7.9966) (32.2297, 7.9999) (32.2099, 8.0031) (32.1903, 8.0063) (32.1706, 8.0095) (32.151, 8.0126) (32.1315, 8.0157) (32.112, 8.0188) (32.0925, 8.0218) (32.0731, 8.0248) (32.0537, 8.0277) (32.0343, 8.0306) (32.015, 8.0335) (31.9957, 8.0363) (31.9765, 8.0391) (31.9573, 8.0419) (31.9382, 8.0446) (31.9191, 8.0473) (31.9, 8.0499) (31.881, 8.0525) (31.862, 8.0551) (31.8431, 8.0577) (31.8242, 8.0602) (31.8054, 8.0626) (31.7866, 8.0651) (31.7678, 8.0675) (31.7491, 8.0698) (31.7304, 8.0722) (31.7118, 8.0745) (31.6932, 8.0767) (31.6747, 8.0789) (31.6562, 8.0811) (31.6378, 8.0833) (31.6194, 8.0854) (31.601, 8.0875) (31.5828, 8.0895) (31.5645, 8.0915) (31.5463, 8.0935) (31.5281, 8.0955) (31.51, 8.0974) (31.492, 8.0993) (31.4739, 8.1011) (31.456, 8.1029) (31.4381, 8.1047) (31.4202, 8.1064) (31.4024, 8.1081) (31.3846, 8.1098) (31.3669, 8.1114) (31.3492, 8.113) (31.3316, 8.1146) (31.314, 8.1161) (31.2965, 8.1176) (31.279, 8.1191) (31.2616, 8.1205) (31.2442, 8.1219) (31.2269, 8.1233) (31.2097, 8.1247) (31.1924, 8.126) (31.1753, 8.1272) (31.1582, 8.1285) (31.1411, 8.1297) (31.1241, 8.1309) (31.1072, 8.132) (31.0903, 8.1331) (31.0734, 8.1342) (31.0567, 8.1353) (31.0399, 8.1363) (31.0233, 8.1373) (31.0066, 8.1382) (30.9901, 8.1391) (30.9736, 8.14) (30.9571, 8.1409) (30.9407, 8.1417) (30.9244, 8.1425) (30.9081, 8.1433) (30.8919, 8.144) (30.8757, 8.1447) (30.8596, 8.1454) (30.8436, 8.1461) (30.8276, 8.1467) (30.8116, 8.1473) (30.7958, 8.1479) (30.78, 8.1484) (30.7642, 8.1489) (30.7485, 8.1494) (30.7329, 8.1498) (30.7173, 8.1502) (30.7018, 8.1506) (30.6864, 8.151) (30.671, 8.1513) (30.6557, 8.1516) (30.6404, 8.1519) (30.6252, 8.1521) (30.6101, 8.1523) (30.595, 8.1525) (30.58, 8.1527) (30.5651, 8.1528) (30.5502, 8.1529) (30.5354, 8.153) (30.5207, 8.1531) (30.506, 8.1531) (30.4914, 8.1531) (30.4769, 8.1531) (30.4624, 8.153) (30.448, 8.153) (30.4337, 8.1529) (30.4194, 8.1527) (30.4052, 8.1526) (30.3911, 8.1524) (30.377, 8.1522) (30.363, 8.152) (30.3491, 8.1517) (30.3353, 8.1515) (30.3215, 8.1512) (30.3078, 8.1509) (30.2942, 8.1505) (30.2806, 8.1501) (30.2671, 8.1498) (30.2537, 8.1493) (30.2404, 8.1489) (30.2272, 8.1485) (30.214, 8.148) (30.2009, 8.1475) (30.1879, 8.1469) (30.1749, 8.1464) (30.162, 8.1458) (30.1493, 8.1453) (30.1365, 8.1446) (30.1239, 8.144) (30.1114, 8.1434) (30.0989, 8.1427) (30.0865, 8.142) (30.0742, 8.1413) (30.062, 8.1406) (30.0498, 8.1399) (30.0378, 8.1391) (30.0258, 8.1383) (30.0139, 8.1375) (30.0021, 8.1367) (29.9904, 8.1359) (29.9787, 8.135) (29.9672, 8.1342) (29.9557, 8.1333) (29.9443, 8.1324) (29.9331, 8.1315) (29.9219, 8.1305) (29.9108, 8.1296) (29.8998, 8.1286) (29.8888, 8.1277) (29.878, 8.1267) (29.8673, 8.1257) (29.8567, 8.1247) (29.8461, 8.1237) (29.8357, 8.1226) (29.8253, 8.1216) (29.8151, 8.1205) (29.8049, 8.1194) (29.7949, 8.1184) (29.7849, 8.1173) (29.775, 8.1162) (29.7653, 8.1151) (29.7556, 8.1139) (29.7461, 8.1128) (29.7367, 8.1117) (29.7273, 8.1105) (29.7181, 8.1094) (29.709, 8.1082) (29.6999, 8.1071) (29.691, 8.1059) (29.6822, 8.1047) (29.6736, 8.1036) (29.665, 8.1024) (29.6565, 8.1012) (29.6482, 8.1) (29.6399, 8.0988) (29.6318, 8.0976) (29.6238, 8.0965) (29.616, 8.0953) (29.6082, 8.0941) (29.6006, 8.0929) (29.5931, 8.0917) (29.5857, 8.0905) (29.5784, 8.0893) (29.5713, 8.0882) (29.5643, 8.087) (29.5574, 8.0858) (29.5507, 8.0847) (29.5441, 8.0835) (29.5376, 8.0824) (29.5313, 8.0812) (29.5251, 8.0801) (29.519, 8.079) (29.5131, 8.0779) (29.5073, 8.0768) (29.5017, 8.0757) (29.4962, 8.0747) (29.4909, 8.0736) (29.4857, 8.0726) (29.4807, 8.0716) (29.4758, 8.0706) (29.4711, 8.0696) (29.4666, 8.0687) (29.4622, 8.0677) (29.458, 8.0668) (29.4539, 8.066) (29.45, 8.0651) (29.4463, 8.0643) (29.4428, 8.0635) (29.4395, 8.0627) (29.4363, 8.062) (29.4333, 8.0613) (29.4305, 8.0606) (29.4279, 8.06) (29.4255, 8.0594) (29.4233, 8.0589) (29.4213, 8.0584) (29.4195, 8.0579) (29.4179, 8.0575) (29.4166, 8.0572) (29.4157, 8.057) (29.4151, 8.0568) (29.4148, 8.0567) (29.4146, 8.0567) knots -1 -1 -1 -1 -1 -1 -0.99583333 -0.99166667 -0.9875 -0.98333333 -0.97916667 -0.975 -0.97083333 -0.96666667 -0.9625 -0.95833333 -0.95416667 -0.95 -0.94583333 -0.94166667 -0.9375 -0.93333333 -0.92916667 -0.925 -0.92083333 -0.91666667 -0.9125 -0.90833333 -0.90416667 -0.9 -0.89583333 -0.89166667 -0.8875 -0.88333333 -0.87916667 -0.875 -0.87083333 -0.86666667 -0.8625 -0.85833333 -0.85416667 -0.85 -0.84583333 -0.84166667 -0.8375 -0.83333333 -0.82916667 -0.825 -0.82083333 -0.81666667 -0.8125 -0.80833333 -0.80416667 -0.8 -0.79583333 -0.79166667 -0.7875 -0.78333333 -0.77916667 -0.775 -0.77083333 -0.76666667 -0.7625 -0.75833333 -0.75416667 -0.75 -0.74583333 -0.74166667 -0.7375 -0.73333333 -0.72916667 -0.725 -0.72083333 -0.71666667 -0.7125 -0.70833333 -0.70416667 -0.7 -0.69583333 -0.69166667 -0.6875 -0.68333333 -0.67916667 -0.675 -0.67083333 -0.66666667 -0.6625 -0.65833333 -0.65416667 -0.65 -0.64583333 -0.64166667 -0.6375 -0.63333333 -0.62916667 -0.625 -0.62083333 -0.61666667 -0.6125 -0.60833333 -0.60416667 -0.6 -0.59583333 -0.59166667 -0.5875 -0.58333333 -0.57916667 -0.575 -0.57083333 -0.56666667 -0.5625 -0.55833333 -0.55416667 -0.55 -0.54583333 -0.54166667 -0.5375 -0.53333333 -0.52916667 -0.525 -0.52083333 -0.51666667 -0.5125 -0.50833333 -0.50416667 -0.5 -0.49583333 -0.49166667 -0.4875 -0.48333333 -0.47916667 -0.475 -0.47083333 -0.46666667 -0.4625 -0.45833333 -0.45416667 -0.45 -0.44583333 -0.44166667 -0.4375 -0.43333333 -0.42916667 -0.425 -0.42083333 -0.41666667 -0.4125 -0.40833333 -0.40416667 -0.4 -0.39583333 -0.39166667 -0.3875 -0.38333333 -0.37916667 -0.375 -0.37083333 -0.36666667 -0.3625 -0.35833333 -0.35416667 -0.35 -0.34583333 -0.34166667 -0.3375 -0.33333333 -0.32916667 -0.325 -0.32083333 -0.31666667 -0.3125 -0.30833333 -0.30416667 -0.3 -0.29583333 -0.29166667 -0.2875 -0.28333333 -0.27916667 -0.275 -0.27083333 -0.26666667 -0.2625 -0.25833333 -0.25416667 -0.25 -0.24583333 -0.24166667 -0.2375 -0.23333333 -0.22916667 -0.225 -0.22083333 -0.21666667 -0.2125 -0.20833333 -0.20416667 -0.2 -0.19583333 -0.19166667 -0.1875 -0.18333333 -0.17916667 -0.175 -0.17083333 -0.16666667 -0.1625 -0.15833333 -0.15416667 -0.15 -0.14583333 -0.14166667 -0.1375 -0.13333333 -0.12916667 -0.125 -0.12083333 -0.11666667 -0.1125 -0.10833333 -0.10416667 -0.1 -0.09583333 -0.09166667 -0.0875 -0.08333333 -0.07916667 -0.075 -0.07083333 -0.06666667 -0.0625 -0.05833333 -0.05416667 -0.05 -0.04583333 -0.04166667 -0.0375 -0.03333333 -0.02916667 -0.025 -0.02083333 -0.01666667 -0.0125 -0.00833333 -0.00416667 0 0 0 0 0 0
  line L66 (29.4146, 8.0567) -> (29.4133, 8.0563)
  line L67 (29.4133, 8.0563) -> (27.8492, 7.6279)
  arc A34 (27.8492, 7.6279) -> (27.0141, 10.1982) centre (0, 0) ccw
  line L68 (27.0141, 10.1982) -> (28.5312, 10.771)
  line L69 (28.5312, 10.771) -> (28.5325, 10.7715)
  spline S34 degree 5 poles (28.5325, 10.7715) (28.5327, 10.7715) (28.533, 10.7717) (28.5336, 10.7719) (28.5344, 10.7722) (28.5357, 10.7727) (28.5372, 10.7733) (28.5389, 10.774) (28.5409, 10.7748) (28.543, 10.7757) (28.5452, 10.7766) (28.5477, 10.7776) (28.5504, 10.7787) (28.5532, 10.7799) (28.5562, 10.7812) (28.5593, 10.7826) (28.5626, 10.784) (28.5661, 10.7855) (28.5698, 10.7871) (28.5736, 10.7888) (28.5775, 10.7905) (28.5816, 10.7923) (28.5858, 10.7942) (28.5902, 10.7962) (28.5947, 10.7983) (28.5994, 10.8004) (28.6042, 10.8026) (28.6091, 10.8049) (28.6142, 10.8073) (28.6194, 10.8097) (28.6247, 10.8122) (28.6301, 10.8148) (28.6357, 10.8175) (28.6413, 10.8202) (28.6471, 10.823) (28.653, 10.8259) (28.6591, 10.8288) (28.6652, 10.8318) (28.6714, 10.8349) (28.6778, 10.8381) (28.6842, 10.8414) (28.6908, 10.8447) (28.6975, 10.848) (28.7043, 10.8515) (28.7111, 10.855) (28.7181, 10.8586) (28.7252, 10.8623) (28.7323, 10.866) (28.7396, 10.8698) (28.747, 10.8737) (28.7544, 10.8777) (28.7619, 10.8817) (28.7696, 10.8858) (28.7773, 10.8899) (28.7851, 10.8941) (28.793, 10.8984) (28.801, 10.9028) (28.809, 10.9072) (28.8172, 10.9117) (28.8254, 10.9163) (28.8337, 10.9209) (28.8421, 10.9256) (28.8505, 10.9304) (28.8591, 10.9352) (28.8677, 10.9401) (28.8764, 10.9451) (28.8852, 10.9501) (28.894, 10.9552) (28.9029, 10.9604) (28.9119, 10.9656) (28.921, 10.9709) (28.9301, 10.9763) (28.9393, 10.9817) (28.9486, 10.9872) (28.9579, 10.9928) (28.9673, 10.9984) (28.9768, 11.0041) (28.9863, 11.0099) (28.9959, 11.0157) (29.0056, 11.0216) (29.0153, 11.0276) (29.0251, 11.0336) (29.0349, 11.0397) (29.0449, 11.0458) (29.0548, 11.052) (29.0649, 11.0583) (29.0749, 11.0647) (29.0851, 11.0711) (29.0953, 11.0776) (29.1056, 11.0841) (29.1159, 11.0907) (29.1262, 11.0974) (29.1367, 11.1041) (29.1472, 11.1109) (29.1577, 11.1177) (29.1683, 11.1247) (29.1789, 11.1316) (29.1896, 11.1387) (29.2004, 11.1458) (29.2111, 11.153) (29.222, 11.1602) (29.2329, 11.1675) (29.2438, 11.1748) (29.2548, 11.1823) (29.2659, 11.1897) (29.2769, 11.1973) (29.2881, 11.2049) (29.2993, 11.2126) (29.3105, 11.2203) (29.3217, 11.2281) (29.3331, 11.2359) (29.3444, 11.2439) (29.3558, 11.2518) (29.3673, 11.2599) (29.3788, 11.268) (29.3903, 11.2761) (29.4019, 11.2844) (29.4135, 11.2926) (29.4251, 11.301) (29.4368, 11.3094) (29.4486, 11.3179) (29.4603, 11.3264) (29.4721, 11.335) (29.484, 11.3436) (29.4959, 11.3523) (29.5078, 11.3611) (29.5198, 11.3699) (29.5318, 11.3788) (29.5438, 11.3878) (29.5559, 11.3968) (29.568, 11.4059) (29.5802, 11.415) (29.5923, 11.4242) (29.6046, 11.4334) (29.6168, 11.4427) (29.6291, 11.4521) (29.6414, 11.4615) (29.6538, 11.471) (29.6661, 11.4806) (29.6786, 11.4902) (29.691, 11.4998) (29.7035, 11.5095) (29.716, 11.5193) (29.7285, 11.5292) (29.7411, 11.5391) (29.7537, 11.549) (29.7663, 11.559) (29.779, 11.5691) (29.7917, 11.5793) (29.8044, 11.5895) (29.8172, 11.5997) (29.8299, 11.61) (29.8427, 11.6204) (29.8556, 11.6308) (29.8684, 11.6413) (29.8813, 11.6518) (29.8942, 11.6624) (29.9071, 11.6731) (29.9201, 11.6838) (29.9331, 11.6946) (29.9461, 11.7054) (29.9591, 11.7163) (29.9722, 11.7272) (29.9853, 11.7382) (29.9984, 11.7493) (30.0115, 11.7604) (30.0247, 11.7716) (30.0379, 11.7828) (30.0511, 11.7941) (30.0643, 11.8055) (30.0775, 11.8169) (30.0908, 11.8283) (30.1041, 11.8398) (30.1174, 11.8514) (30.1308, 11.863) (30.1441, 11.8747) (30.1575, 11.8865) (30.1709, 11.8982) (30.1843, 11.9101) (30.1977, 11.922) (30.2112, 11.934) (30.2247, 11.946) (30.2382, 11.9581) (30.2517, 11.9702) (30.2652, 11.9824) (30.2787, 11.9946) (30.2923, 12.0069) (30.3059, 12.0193) (30.3195, 12.0317) (30.3331, 12.0442) (30.3467, 12.0567) (30.3604, 12.0693) (30.3741, 12.0819) (30.3877, 12.0946) (30.4014, 12.1074) (30.4152, 12.1202) (30.4289, 12.133) (30.4426, 12.1459) (30.4564, 12.1589) (30.4702, 12.1719) (30.484, 12.185) (30.4978, 12.1981) (30.5116, 12.2113) (30.5254, 12.2245) (30.5393, 12.2378) (30.5531, 12.2512) (30.567, 12.2646) (30.5809, 12.278) (30.5948, 12.2915) (30.6087, 12.3051) (30.6226, 12.3187) (30.6366, 12.3324) (30.6505, 12.3461) (30.6645, 12.3599) (30.6785, 12.3737) (30.6924, 12.3876) (30.7064, 12.4016) (30.7204, 12.4155) (30.7345, 12.4296) (30.7485, 12.4437) (30.7625, 12.4579) (30.7766, 12.4721) (30.7906, 12.4863) (30.8047, 12.5006) (30.8188, 12.515) (30.8328, 12.5294) (30.8469, 12.5439) (30.861, 12.5584) (30.8752, 12.573) (30.8893, 12.5876) (30.9034, 12.6023) (30.9175, 12.6171) (30.9317, 12.6319) (30.9458, 12.6467) (30.96, 12.6616) (30.9742, 12.6765) (30.9883, 12.6916) (31.0025, 12.7066) (31.0167, 12.7217) (31.0309, 12.7369) (31.0451, 12.7521) (31.0565, 12.7643) (31.065, 12.7735) (31.0707, 12.7796) (31.0735, 12.7827) knots 0 0 0 0 0 0 0.00416667 0.00833333 0.0125 0.01666667 0.02083333 0.025 0.02916667 0.03333333 0.0375 0.04166667 0.04583333 0.05 0.05416667 0.05833333 0.0625 0.06666667 0.07083333 0.075 0.07916667 0.08333333 0.0875 0.09166667 0.09583333 0.1 0.10416667 0.10833333 0.1125 0.11666667 0.12083333 0.125 0.12916667 0.13333333 0.1375 0.14166667 0.14583333 0.15 0.15416667 0.15833333 0.1625 0.16666667 0.17083333 0.175 0.17916667 0.18333333 0.1875 0.19166667 0.19583333 0.2 0.20416667 0.20833333 0.2125 0.21666667 0.22083333 0.225 0.22916667 0.23333333 0.2375 0.24166667 0.24583333 0.25 0.25416667 0.25833333 0.2625 0.26666667 0.27083333 0.275 0.27916667 0.28333333 0.2875 0.29166667 0.29583333 0.3 0.30416667 0.30833333 0.3125 0.31666667 0.32083333 0.325 0.32916667 0.33333333 0.3375 0.34166667 0.34583333 0.35 0.35416667 0.35833333 0.3625 0.36666667 0.37083333 0.375 0.37916667 0.38333333 0.3875 0.39166667 0.39583333 0.4 0.40416667 0.40833333 0.4125 0.41666667 0.42083333 0.425 0.42916667 0.43333333 0.4375 0.44166667 0.44583333 0.45 0.45416667 0.45833333 0.4625 0.46666667 0.47083333 0.475 0.47916667 0.48333333 0.4875 0.49166667 0.49583333 0.5 0.50416667 0.50833333 0.5125 0.51666667 0.52083333 0.525 0.52916667 0.53333333 0.5375 0.54166667 0.54583333 0.55 0.55416667 0.55833333 0.5625 0.56666667 0.57083333 0.575 0.57916667 0.58333333 0.5875 0.59166667 0.59583333 0.6 0.60416667 0.60833333 0.6125 0.61666667 0.62083333 0.625 0.62916667 0.63333333 0.6375 0.64166667 0.64583333 0.65 0.65416667 0.65833333 0.6625 0.66666667 0.67083333 0.675 0.67916667 0.68333333 0.6875 0.69166667 0.69583333 0.7 0.70416667 0.70833333 0.7125 0.71666667 0.72083333 0.725 0.72916667 0.73333333 0.7375 0.74166667 0.74583333 0.75 0.75416667 0.75833333 0.7625 0.76666667 0.77083333 0.775 0.77916667 0.78333333 0.7875 0.79166667 0.79583333 0.8 0.80416667 0.80833333 0.8125 0.81666667 0.82083333 0.825 0.82916667 0.83333333 0.8375 0.84166667 0.84583333 0.85 0.85416667 0.85833333 0.8625 0.86666667 0.87083333 0.875 0.87916667 0.88333333 0.8875 0.89166667 0.89583333 0.9 0.90416667 0.90833333 0.9125 0.91666667 0.92083333 0.925 0.92916667 0.93333333 0.9375 0.94166667 0.94583333 0.95 0.95416667 0.95833333 0.9625 0.96666667 0.97083333 0.975 0.97916667 0.98333333 0.9875 0.99166667 0.99583333 1 1 1 1 1 1
  arc A35 (31.0735, 12.7827) -> (30.2916, 14.5388) centre (0, 0) ccw
  spline S35 degree 5 poles (30.2916, 14.5388) (30.2874, 14.5388) (30.2791, 14.5387) (30.2665, 14.5385) (30.2499, 14.5382) (30.2291, 14.5378) (30.2083, 14.5374) (30.1876, 14.537) (30.1669, 14.5365) (30.1463, 14.536) (30.1257, 14.5355) (30.1051, 14.5349) (30.0846, 14.5344) (30.0642, 14.5337) (30.0438, 14.5331) (30.0234, 14.5324) (30.0031, 14.5317) (29.9828, 14.531) (29.9626, 14.5302) (29.9424, 14.5294) (29.9222, 14.5286) (29.9021, 14.5278) (29.8821, 14.5269) (29.8621, 14.526) (29.8421, 14.5251) (29.8222, 14.5241) (29.8024, 14.5231) (29.7825, 14.5221) (29.7628, 14.5211) (29.743, 14.52) (29.7234, 14.5189) (29.7037, 14.5178) (29.6842, 14.5166) (29.6646, 14.5154) (29.6451, 14.5142) (29.6257, 14.513) (29.6063, 14.5117) (29.587, 14.5104) (29.5677, 14.5091) (29.5484, 14.5078) (29.5292, 14.5064) (29.5101, 14.505) (29.491, 14.5036) (29.472, 14.5021) (29.453, 14.5007) (29.434, 14.4992) (29.4151, 14.4976) (29.3963, 14.4961) (29.3775, 14.4945) (29.3587, 14.4929) (29.3401, 14.4913) (29.3214, 14.4896) (29.3028, 14.4879) (29.2843, 14.4862) (29.2658, 14.4845) (29.2474, 14.4828) (29.229, 14.481) (29.2107, 14.4792) (29.1924, 14.4774) (29.1742, 14.4755) (29.156, 14.4736) (29.1379, 14.4717) (29.1199, 14.4698) (29.1019, 14.4679) (29.0839, 14.4659) (29.066, 14.4639) (29.0482, 14.4619) (29.0304, 14.4598) (29.0126, 14.4578) (28.995, 14.4557) (28.9774, 14.4536) (28.9598, 14.4515) (28.9423, 14.4493) (28.9248, 14.4471) (28.9074, 14.445) (28.8901, 14.4427) (28.8728, 14.4405) (28.8556, 14.4382) (28.8384, 14.436) (28.8213, 14.4337) (28.8043, 14.4313) (28.7873, 14.429) (28.7704, 14.4266) (28.7535, 14.4243) (28.7367, 14.4219) (28.7199, 14.4194) (28.7032, 14.417) (28.6866, 14.4145) (28.67, 14.412) (28.6535, 14.4095) (28.637, 14.407) (28.6206, 14.4045) (28.6043, 14.4019) (28.588, 14.3993) (28.5718, 14.3967) (28.5557, 14.3941) (28.5396, 14.3915) (28.5236, 14.3889) (28.5076, 14.3862) (28.4917, 14.3835) (28.4759, 14.3808) (28.4601, 14.3781) (28.4444, 14.3754) (28.4288, 14.3726) (28.4132, 14.3698) (28.3977, 14.367) (28.3822, 14.3643) (28.3669, 14.3614) (28.3515, 14.3586) (28.3363, 14.3558) (28.3211, 14.3529) (28.306, 14.35) (28.291, 14.3471) (28.276, 14.3442) (28.2611, 14.3413) (28.2462, 14.3384) (28.2314, 14.3354) (28.2167, 14.3325) (28.2021, 14.3295) (28.1875, 14.3265) (28.173, 14.3235) (28.1586, 14.3205) (28.1442, 14.3175) (28.13, 14.3145) (28.1157, 14.3114) (28.1016, 14.3084) (28.0875, 14.3053) (28.0735, 14.3022) (28.0596, 14.2991) (28.0457, 14.296) (28.032, 14.2929) (28.0183, 14.2898) (28.0046, 14.2867) (27.9911, 14.2835) (27.9776, 14.2804) (27.9642, 14.2772) (27.9508, 14.2741) (27.9376, 14.2709) (27.9244, 14.2677) (27.9113, 14.2646) (27.8983, 14.2614) (27.8853, 14.2582) (27.8725, 14.255) (27.8597, 14.2518) (27.847, 14.2485) (27.8343, 14.2453) (27.8218, 14.2421) (27.8093, 14.2389) (27.7969, 14.2356) (27.7846, 14.2324) (27.7724, 14.2292) (27.7602, 14.2259) (27.7482, 14.2227) (27.7362, 14.2194) (27.7243, 14.2162) (27.7125, 14.2129) (27.7008, 14.2097) (27.6891, 14.2064) (27.6776, 14.2032) (27.6661, 14.1999) (27.6547, 14.1967) (27.6435, 14.1934) (27.6323, 14.1902) (27.6211, 14.1869) (27.6101, 14.1837) (27.5992, 14.1804) (27.5883, 14.1772) (27.5776, 14.174) (27.5669, 14.1707) (27.5563, 14.1675) (27.5459, 14.1643) (27.5355, 14.1611) (27.5252, 14.1579) (27.515, 14.1547) (27.5049, 14.1515) (27.4949, 14.1483) (27.485, 14.1451) (27.4752, 14.142) (27.4655, 14.1388) (27.4559, 14.1357) (27.4464, 14.1325) (27.4369, 14.1294) (27.4276, 14.1263) (27.4184, 14.1232) (27.4093, 14.1201) (27.4003, 14.117) (27.3914, 14.114) (27.3826, 14.1109) (27.374, 14.1079) (27.3654, 14.1049) (27.3569, 14.1019) (27.3485, 14.0989) (27.3403, 14.096) (27.3322, 14.093) (27.3241, 14.0901) (27.3162, 14.0872) (27.3084, 14.0843) (27.3007, 14.0815) (27.2931, 14.0787) (27.2857, 14.0759) (27.2784, 14.0731) (27.2711, 14.0703) (27.264, 14.0676) (27.2571, 14.0649) (27.2502, 14.0623) (27.2435, 14.0596) (27.2369, 14.057) (27.2304, 14.0545) (27.224, 14.0519) (27.2178, 14.0494) (27.2117, 14.047) (27.2058, 14.0445) (27.1999, 14.0422) (27.1942, 14.0398) (27.1887, 14.0375) (27.1833, 14.0352) (27.178, 14.033) (27.1728, 14.0308) (27.1679, 14.0287) (27.163, 14.0266) (27.1583, 14.0246) (27.1537, 14.0226) (27.1493, 14.0207) (27.1451, 14.0188) (27.141, 14.017) (27.1371, 14.0152) (27.1333, 14.0135) (27.1297, 14.0119) (27.1262, 14.0103) (27.1229, 14.0088) (27.1198, 14.0073) (27.1169, 14.006) (27.1141, 14.0047) (27.1115, 14.0034) (27.1091, 14.0023) (27.1068, 14.0012) (27.1048, 14.0002) (27.1029, 13.9993) (27.1013, 13.9985) (27.0998, 13.9978) (27.0986, 13.9972) (27.0977, 13.9968) (27.0972, 13.9965) (27.0969, 13.9963) (27.0967, 13.9963) knots -1 -1 -1 -1 -1 -1 -0.99583333 -0.99166667 -0.9875 -0.98333333 -0.97916667 -0.975 -0.97083333 -0.96666667 -0.9625 -0.95833333 -0.95416667 -0.95 -0.94583333 -0.94166667 -0.9375 -0.93333333 -0.92916667 -0.925 -0.92083333 -0.91666667 -0.9125 -0.90833333 -0.90416667 -0.9 -0.89583333 -0.89166667 -0.8875 -0.88333333 -0.87916667 -0.875 -0.87083333 -0.86666667 -0.8625 -0.85833333 -0.85416667 -0.85 -0.84583333 -0.84166667 -0.8375 -0.83333333 -0.82916667 -0.825 -0.82083333 -0.81666667 -0.8125 -0.80833333 -0.80416667 -0.8 -0.79583333 -0.79166667 -0.7875 -0.78333333 -0.77916667 -0.775 -0.77083333 -0.76666667 -0.7625 -0.75833333 -0.75416667 -0.75 -0.74583333 -0.74166667 -0.7375 -0.73333333 -0.72916667 -0.725 -0.72083333 -0.71666667 -0.7125 -0.70833333 -0.70416667 -0.7 -0.69583333 -0.69166667 -0.6875 -0.68333333 -0.67916667 -0.675 -0.67083333 -0.66666667 -0.6625 -0.65833333 -0.65416667 -0.65 -0.64583333 -0.64166667 -0.6375 -0.63333333 -0.62916667 -0.625 -0.62083333 -0.61666667 -0.6125 -0.60833333 -0.60416667 -0.6 -0.59583333 -0.59166667 -0.5875 -0.58333333 -0.57916667 -0.575 -0.57083333 -0.56666667 -0.5625 -0.55833333 -0.55416667 -0.55 -0.54583333 -0.54166667 -0.5375 -0.53333333 -0.52916667 -0.525 -0.52083333 -0.51666667 -0.5125 -0.50833333 -0.50416667 -0.5 -0.49583333 -0.49166667 -0.4875 -0.48333333 -0.47916667 -0.475 -0.47083333 -0.46666667 -0.4625 -0.45833333 -0.45416667 -0.45 -0.44583333 -0.44166667 -0.4375 -0.43333333 -0.42916667 -0.425 -0.42083333 -0.41666667 -0.4125 -0.40833333 -0.40416667 -0.4 -0.39583333 -0.39166667 -0.3875 -0.38333333 -0.37916667 -0.375 -0.37083333 -0.36666667 -0.3625 -0.35833333 -0.35416667 -0.35 -0.34583333 -0.34166667 -0.3375 -0.33333333 -0.32916667 -0.325 -0.32083333 -0.31666667 -0.3125 -0.30833333 -0.30416667 -0.3 -0.29583333 -0.29166667 -0.2875 -0.28333333 -0.27916667 -0.275 -0.27083333 -0.26666667 -0.2625 -0.25833333 -0.25416667 -0.25 -0.24583333 -0.24166667 -0.2375 -0.23333333 -0.22916667 -0.225 -0.22083333 -0.21666667 -0.2125 -0.20833333 -0.20416667 -0.2 -0.19583333 -0.19166667 -0.1875 -0.18333333 -0.17916667 -0.175 -0.17083333 -0.16666667 -0.1625 -0.15833333 -0.15416667 -0.15 -0.14583333 -0.14166667 -0.1375 -0.13333333 -0.12916667 -0.125 -0.12083333 -0.11666667 -0.1125 -0.10833333 -0.10416667 -0.1 -0.09583333 -0.09166667 -0.0875 -0.08333333 -0.07916667 -0.075 -0.07083333 -0.06666667 -0.0625 -0.05833333 -0.05416667 -0.05 -0.04583333 -0.04166667 -0.0375 -0.03333333 -0.02916667 -0.025 -0.02083333 -0.01666667 -0.0125 -0.00833333 -0.00416667 0 0 0 0 0 0
  line L70 (27.0967, 13.9963) -> (27.0955, 13.9956)
  line L71 (27.0955, 13.9956) -> (25.6547, 13.2514)
  arc A36 (25.6547, 13.2514) -> (24.3034, 15.5919) centre (0, 0) ccw
  line L72 (24.3034, 15.5919) -> (25.6683, 16.4676)
  line L73 (25.6683, 16.4676) -> (25.6695, 16.4683)